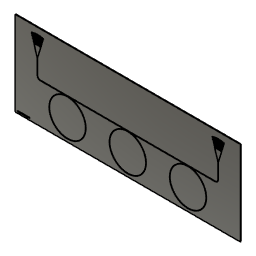
MultiRes (Autodesk Fusion 360 design; units mm, degrees)
Autodesk Fusion 360 part; units mm, degrees
sketch "Sketch1" plane through (0, 0, 0) normal (0, 1, 0) x (1, 0, 0)
  circle A0 centre (0, 0) radius 30
  circle A1 centre (0, 0) radius 30.5
  line L0 (-45, -30.95) -> (45, -30.95)
  line L1 (-50, -35.95) -> (-50, -60.95)
  arc A2 (-45, -30.95) -> (-50, -35.95) centre (-45, -35.95) ccw
  line L2 (-45, -31.2) -> (45, -31.2)
  arc A3 (-45, -31.2) -> (-49.75, -35.95) centre (-45, -35.95) ccw
  line L3 (-49.75, -35.95) -> (-49.75, -60.95)
  line L4 (-45, -30.7) -> (45, -30.7)
  arc A4 (-45, -30.7) -> (-50.25, -35.95) centre (-45, -35.95) ccw
  line L5 (-50.25, -35.95) -> (-50.25, -60.95)
  line L6 (-50.25, -60.95) -> (-49.75, -60.95)
  line L7 (-49.75, -60.95) -> (-39.9666, -92.95)
  line L8 (-50.25, -60.95) -> (-60.0334, -92.95)
  arc A5 (-60.0334, -92.95) -> (-39.9666, -92.95) centre (-50, -60.95) ccw
  arc A6 (-55.6371, -78.5703) -> (-44.3629, -78.5703) centre (-50, -60.95) ccw
  arc A7 (-55.698, -78.7608) -> (-44.302, -78.7608) centre (-50, -60.95) ccw
  arc A8 (-55.7589, -78.9512) -> (-44.2411, -78.9512) centre (-50, -60.95) ccw
  arc A9 (-55.8199, -79.1417) -> (-44.1801, -79.1417) centre (-50, -60.95) ccw
  arc A10 (-55.9722, -79.618) -> (-44.0278, -79.618) centre (-50, -60.95) ccw
  arc A11 (-56.0332, -79.8084) -> (-43.9668, -79.8084) centre (-50, -60.95) ccw
  arc A12 (-56.0941, -79.9989) -> (-43.9059, -79.9989) centre (-50, -60.95) ccw
  arc A13 (-56.1551, -80.1894) -> (-43.8449, -80.1894) centre (-50, -60.95) ccw
  arc A14 (-56.3074, -80.6656) -> (-43.6926, -80.6656) centre (-50, -60.95) ccw
  arc A15 (-56.3683, -80.8561) -> (-43.6317, -80.8561) centre (-50, -60.95) ccw
  arc A16 (-56.4293, -81.0466) -> (-43.5707, -81.0466) centre (-50, -60.95) ccw
  arc A17 (-56.4902, -81.2371) -> (-43.5098, -81.2371) centre (-50, -60.95) ccw
  arc A18 (-56.6426, -81.7133) -> (-43.3574, -81.7133) centre (-50, -60.95) ccw
  arc A19 (-56.7035, -81.9038) -> (-43.2965, -81.9038) centre (-50, -60.95) ccw
  arc A20 (-56.7645, -82.0943) -> (-43.2355, -82.0943) centre (-50, -60.95) ccw
  arc A21 (-56.8254, -82.2848) -> (-43.1746, -82.2848) centre (-50, -60.95) ccw
  arc A22 (-56.9778, -82.761) -> (-43.0222, -82.761) centre (-50, -60.95) ccw
  arc A23 (-57.0387, -82.9515) -> (-42.9613, -82.9515) centre (-50, -60.95) ccw
  arc A24 (-57.0996, -83.142) -> (-42.9004, -83.142) centre (-50, -60.95) ccw
  arc A25 (-57.1606, -83.3325) -> (-42.8394, -83.3325) centre (-50, -60.95) ccw
  arc A26 (-57.3129, -83.8087) -> (-42.6871, -83.8087) centre (-50, -60.95) ccw
  arc A27 (-57.3739, -83.9992) -> (-42.6261, -83.9992) centre (-50, -60.95) ccw
  arc A28 (-57.4348, -84.1897) -> (-42.5652, -84.1897) centre (-50, -60.95) ccw
  arc A29 (-57.4958, -84.3802) -> (-42.5042, -84.3802) centre (-50, -60.95) ccw
  arc A30 (-57.6481, -84.8564) -> (-42.3519, -84.8564) centre (-50, -60.95) ccw
  arc A31 (-57.7091, -85.0469) -> (-42.2909, -85.0469) centre (-50, -60.95) ccw
  arc A32 (-57.77, -85.2374) -> (-42.23, -85.2374) centre (-50, -60.95) ccw
  arc A33 (-57.8309, -85.4279) -> (-42.1691, -85.4279) centre (-50, -60.95) ccw
  arc A34 (-57.9833, -85.9041) -> (-42.0167, -85.9041) centre (-50, -60.95) ccw
  arc A35 (-58.0442, -86.0946) -> (-41.9558, -86.0946) centre (-50, -60.95) ccw
  arc A36 (-58.1052, -86.2851) -> (-41.8948, -86.2851) centre (-50, -60.95) ccw
  arc A37 (-58.1661, -86.4756) -> (-41.8339, -86.4756) centre (-50, -60.95) ccw
  arc A38 (-58.3185, -86.9518) -> (-41.6815, -86.9518) centre (-50, -60.95) ccw
  arc A39 (-58.3794, -87.1423) -> (-41.6206, -87.1423) centre (-50, -60.95) ccw
  arc A40 (-58.4403, -87.3328) -> (-41.5597, -87.3328) centre (-50, -60.95) ccw
  arc A41 (-58.5013, -87.5233) -> (-41.4987, -87.5233) centre (-50, -60.95) ccw
  arc A42 (-58.6536, -87.9995) -> (-41.3464, -87.9995) centre (-50, -60.95) ccw
  arc A43 (-58.7146, -88.19) -> (-41.2854, -88.19) centre (-50, -60.95) ccw
  arc A44 (-58.7755, -88.3805) -> (-41.2245, -88.3805) centre (-50, -60.95) ccw
  arc A45 (-58.8365, -88.571) -> (-41.1635, -88.571) centre (-50, -60.95) ccw
  arc A46 (-58.9888, -89.0472) -> (-41.0112, -89.0472) centre (-50, -60.95) ccw
  arc A47 (-59.0498, -89.2377) -> (-40.9502, -89.2377) centre (-50, -60.95) ccw
  arc A48 (-59.1107, -89.4282) -> (-40.8893, -89.4282) centre (-50, -60.95) ccw
  arc A49 (-59.1716, -89.6186) -> (-40.8284, -89.6186) centre (-50, -60.95) ccw
  arc A50 (-59.324, -90.0949) -> (-40.676, -90.0949) centre (-50, -60.95) ccw
  arc A51 (-59.3849, -90.2854) -> (-40.6151, -90.2854) centre (-50, -60.95) ccw
  arc A52 (-59.4459, -90.4758) -> (-40.5541, -90.4758) centre (-50, -60.95) ccw
  arc A53 (-59.5068, -90.6663) -> (-40.4932, -90.6663) centre (-50, -60.95) ccw
  arc A54 (-59.6592, -91.1426) -> (-40.3408, -91.1426) centre (-50, -60.95) ccw
  arc A55 (-59.7201, -91.333) -> (-40.2799, -91.333) centre (-50, -60.95) ccw
  arc A56 (-59.7811, -91.5235) -> (-40.2189, -91.5235) centre (-50, -60.95) ccw
  arc A57 (-59.842, -91.714) -> (-40.158, -91.714) centre (-50, -60.95) ccw
  arc A58 (-59.9943, -92.1902) -> (-40.0057, -92.1902) centre (-50, -60.95) ccw
  arc A59 (-60.0553, -92.3807) -> (-39.9447, -92.3807) centre (-50, -60.95) ccw
  arc A60 (-60.1162, -92.5712) -> (-39.8838, -92.5712) centre (-50, -60.95) ccw
  arc A61 (-60.1772, -92.7617) -> (-39.8228, -92.7617) centre (-50, -60.95) ccw
  line L9 (-83.2157, 31.3606) -> (-62.7231, 31.3606)
  line L10 (-62.7231, 31.3606) -> (-62.7231, 32.5289)
  line L11 (-62.7231, 32.5289) -> (-83.2157, 32.5289)
  line L12 (-83.2157, 32.5289) -> (-83.2157, 31.3606)
  line L13 (-62.9231, 32.3289) -> (-83.0157, 32.3289)
  line L14 (-83.0157, 32.3289) -> (-83.0157, 31.5606)
  line L15 (-83.0157, 31.5606) -> (-62.9231, 31.5606)
  line L16 (-62.9231, 31.5606) -> (-62.9231, 32.3289)
  line L17 (-73.012, 31.5606) -> (-73.012, 32.3289)
  line L18 (-73.012, 31.5606) -> (-62.9231, 31.5606)
  line L19 (-62.9231, 31.5606) -> (-62.9231, 32.3289)
  line L20 (-62.9231, 32.3289) -> (-73.012, 32.3289)
  line L21 (-73.012, 32.3289) -> (-73.012, 31.5606)
  line L22 (-87.1137, -104.9748) -> (286.8892, -104.9748)
  line L23 (286.8892, -104.9748) -> (286.8892, 35.3192)
  line L24 (286.8892, 35.3192) -> (-87.1137, 35.3192)
  line L25 (-87.1137, 35.3192) -> (-87.1137, -104.9748)
  arc A62 (242.5042, -84.3802) -> (257.4958, -84.3802) centre (250, -60.95) ccw
  arc A63 (243.9668, -79.8084) -> (256.0332, -79.8084) centre (250, -60.95) ccw
  arc A64 (244.302, -78.7608) -> (255.698, -78.7608) centre (250, -60.95) ccw
  arc A65 (243.9059, -79.9989) -> (256.0941, -79.9989) centre (250, -60.95) ccw
  arc A66 (243.2355, -82.0943) -> (256.7645, -82.0943) centre (250, -60.95) ccw
  arc A67 (242.2909, -85.0469) -> (257.7091, -85.0469) centre (250, -60.95) ccw
  arc A68 (243.6317, -80.8561) -> (256.3683, -80.8561) centre (250, -60.95) ccw
  arc A69 (243.6926, -80.6656) -> (256.3074, -80.6656) centre (250, -60.95) ccw
  arc A70 (243.5098, -81.2371) -> (256.4902, -81.2371) centre (250, -60.95) ccw
  arc A71 (242.6261, -83.9992) -> (257.3739, -83.9992) centre (250, -60.95) ccw
  arc A72 (239.9447, -92.3807) -> (260.0553, -92.3807) centre (250, -60.95) ccw
  arc A73 (241.2854, -88.19) -> (258.7146, -88.19) centre (250, -60.95) ccw
  arc A74 (240.5541, -90.4758) -> (259.4459, -90.4758) centre (250, -60.95) ccw
  arc A75 (241.1635, -88.571) -> (258.8365, -88.571) centre (250, -60.95) ccw
  arc A76 (240.2189, -91.5235) -> (259.7811, -91.5235) centre (250, -60.95) ccw
  arc A77 (241.9558, -86.0946) -> (258.0442, -86.0946) centre (250, -60.95) ccw
  arc A78 (242.0167, -85.9041) -> (257.9833, -85.9041) centre (250, -60.95) ccw
  line L26 (249.75, -60.95) -> (239.9666, -92.95)
  line L27 (249.75, -60.95) -> (250.25, -60.95)
  arc A79 (240.3408, -91.1426) -> (259.6592, -91.1426) centre (250, -60.95) ccw
  arc A80 (242.23, -85.2374) -> (257.77, -85.2374) centre (250, -60.95) ccw
  line L28 (250.25, -60.95) -> (260.0334, -92.95)
  arc A81 (240.4932, -90.6663) -> (259.5068, -90.6663) centre (250, -60.95) ccw
  arc A82 (242.1691, -85.4279) -> (257.8309, -85.4279) centre (250, -60.95) ccw
  arc A83 (243.1746, -82.2848) -> (256.8254, -82.2848) centre (250, -60.95) ccw
  arc A84 (244.1801, -79.1417) -> (255.8199, -79.1417) centre (250, -60.95) ccw
  arc A85 (242.6871, -83.8087) -> (257.3129, -83.8087) centre (250, -60.95) ccw
  arc A86 (244.3629, -78.5703) -> (255.6371, -78.5703) centre (250, -60.95) ccw
  arc A87 (243.3574, -81.7133) -> (256.6426, -81.7133) centre (250, -60.95) ccw
  arc A88 (243.8449, -80.1894) -> (256.1551, -80.1894) centre (250, -60.95) ccw
  arc A89 (242.8394, -83.3325) -> (257.1606, -83.3325) centre (250, -60.95) ccw
  arc A90 (240.9502, -89.2377) -> (259.0498, -89.2377) centre (250, -60.95) ccw
  arc A91 (241.6815, -86.9518) -> (258.3185, -86.9518) centre (250, -60.95) ccw
  arc A92 (242.3519, -84.8564) -> (257.6481, -84.8564) centre (250, -60.95) ccw
  arc A93 (242.5652, -84.1897) -> (257.4348, -84.1897) centre (250, -60.95) ccw
  arc A94 (240.676, -90.0949) -> (259.324, -90.0949) centre (250, -60.95) ccw
  arc A95 (244.2411, -78.9512) -> (255.7589, -78.9512) centre (250, -60.95) ccw
  arc A96 (240.6151, -90.2854) -> (259.3849, -90.2854) centre (250, -60.95) ccw
  arc A97 (242.9613, -82.9515) -> (257.0387, -82.9515) centre (250, -60.95) ccw
  arc A98 (239.8228, -92.7617) -> (260.1772, -92.7617) centre (250, -60.95) ccw
  arc A99 (241.8339, -86.4756) -> (258.1661, -86.4756) centre (250, -60.95) ccw
  arc A100 (239.8838, -92.5712) -> (260.1162, -92.5712) centre (250, -60.95) ccw
  arc A101 (242.9004, -83.142) -> (257.0996, -83.142) centre (250, -60.95) ccw
  arc A102 (241.8948, -86.2851) -> (258.1052, -86.2851) centre (250, -60.95) ccw
  arc A103 (243.2965, -81.9038) -> (256.7035, -81.9038) centre (250, -60.95) ccw
  arc A104 (241.2245, -88.3805) -> (258.7755, -88.3805) centre (250, -60.95) ccw
  arc A105 (240.8284, -89.6186) -> (259.1716, -89.6186) centre (250, -60.95) ccw
  arc A106 (240.158, -91.714) -> (259.842, -91.714) centre (250, -60.95) ccw
  arc A107 (240.0057, -92.1902) -> (259.9943, -92.1902) centre (250, -60.95) ccw
  arc A108 (243.0222, -82.761) -> (256.9778, -82.761) centre (250, -60.95) ccw
  arc A109 (239.9666, -92.95) -> (260.0334, -92.95) centre (250, -60.95) ccw
  arc A110 (241.4987, -87.5233) -> (258.5013, -87.5233) centre (250, -60.95) ccw
  arc A111 (244.0278, -79.618) -> (255.9722, -79.618) centre (250, -60.95) ccw
  arc A112 (243.5707, -81.0466) -> (256.4293, -81.0466) centre (250, -60.95) ccw
  arc A113 (241.0112, -89.0472) -> (258.9888, -89.0472) centre (250, -60.95) ccw
  arc A114 (241.5597, -87.3328) -> (258.4403, -87.3328) centre (250, -60.95) ccw
  arc A115 (240.2799, -91.333) -> (259.7201, -91.333) centre (250, -60.95) ccw
  arc A116 (240.8893, -89.4282) -> (259.1107, -89.4282) centre (250, -60.95) ccw
  arc A117 (241.6206, -87.1423) -> (258.3794, -87.1423) centre (250, -60.95) ccw
  arc A118 (241.3464, -87.9995) -> (258.6536, -87.9995) centre (250, -60.95) ccw
  circle A119 centre (100, 0) radius 30.5
  line L29 (55, -30.7) -> (145, -30.7)
  line L30 (55, -30.95) -> (145, -30.95)
  line L31 (55, -31.2) -> (145, -31.2)
  circle A120 centre (100, 0) radius 30
  circle A121 centre (200, 0) radius 30.5
  line L32 (155, -30.7) -> (245, -30.7)
  line L33 (155, -30.95) -> (245, -30.95)
  line L34 (155, -31.2) -> (245, -31.2)
  circle A122 centre (200, 0) radius 30
  line L35 (250, -35.95) -> (250, -60.95)
  line L36 (145, -31.2) -> (155, -31.2)
  line L37 (145, -30.7) -> (155, -30.7)
  line L38 (45, -31.2) -> (55, -31.2)
  line L39 (45, -30.7) -> (55, -30.7)
  arc A123 (250, -35.95) -> (245, -30.95) centre (245, -35.95) ccw
  arc A124 (250.25, -35.95) -> (245, -30.7) centre (245, -35.95) ccw
  line L40 (250.25, -35.95) -> (250.25, -60.95)
  arc A125 (249.75, -35.95) -> (245, -31.2) centre (245, -35.95) ccw
  line L41 (249.75, -35.95) -> (249.75, -60.95)
  point P0 (-50, -30.95)
  point P1 (50, -30.95)
  point P2 (100, 0)
  point P3 (200, 0)
  dimension "d1" = 60
  dimension "d2" = 0.5
  dimension "d3" = 30.95
  dimension "d4" = 50
  dimension "d5" = 50
  dimension "d6" = 30
  dimension "d8" = 5
  dimension "d16" = 107
  dimension "d17" = 107
  dimension "d18" = 32
  dimension "d19" = 32
  dimension "d20" = 18.5
  dimension "d21" = 0.2
  dimension "d22" = 0.4
  dimension "d23" = 0.6
  dimension "d24" = 1.1
  dimension "d25" = 1.3
  dimension "d26" = 1.5
  dimension "d27" = 1.7
  dimension "d28" = 2.2
  dimension "d29" = 2.4
  dimension "d30" = 2.6
  dimension "d31" = 2.8
  dimension "d32" = 3.3
  dimension "d33" = 3.5
  dimension "d34" = 3.7
  dimension "d35" = 3.9
  dimension "d36" = 4.4
  dimension "d37" = 4.6
  dimension "d38" = 4.8
  dimension "d39" = 5
  dimension "d40" = 5.5
  dimension "d41" = 5.7
  dimension "d42" = 5.9
  dimension "d43" = 6.1
  dimension "d44" = 6.6
  dimension "d45" = 6.8
  dimension "d46" = 7
  dimension "d47" = 7.2
  dimension "d48" = 7.7
  dimension "d49" = 7.9
  dimension "d50" = 8.1
  dimension "d51" = 8.3
  dimension "d52" = 8.8
  dimension "d53" = 9
  dimension "d54" = 9.2
  dimension "d55" = 9.4
  dimension "d56" = 9.9
  dimension "d57" = 10.1
  dimension "d58" = 10.3
  dimension "d59" = 10.5
  dimension "d60" = 11
  dimension "d61" = 11.2
  dimension "d62" = 11.4
  dimension "d63" = 11.6
  dimension "d64" = 12.1
  dimension "d65" = 12.3
  dimension "d66" = 12.5
  dimension "d67" = 12.7
  dimension "d68" = 13.2
  dimension "d69" = 13.4
  dimension "d70" = 13.6
  dimension "d71" = 13.8
  dimension "d72" = 14.3
  dimension "d73" = 14.5
  dimension "d74" = 14.7
  dimension "d75" = 14.9
  dimension "d80" = -0.2
  dimension "d88" = 374.0029
  dimension "d89" = 107
  dimension "d90" = 107
  dimension "d91" = 32
  dimension "d92" = 32
  dimension "d95" = 200
  dimension "d96" = 0
  dimension "d97" = 5
  dimension "d98" = 0.25
  dimension "d99" = -0.25
  constraint coincident A0.centre A1.centre
  constraint horizontal L0
  constraint perpendicular L0 L1
  constraint coincident P0 L0
  constraint coincident P0 L1
  constraint tangent L0 A2
  constraint tangent L1 A2
  constraint coincident P1 L0
  constraint perpendicular L3 L6
  constraint coincident L1.end A5.centre
  constraint coincident L8 A6.start
  constraint coincident L7 A6.end
  constraint horizontal L9
  constraint vertical L10
  constraint horizontal L11
  constraint vertical L12
  constraint coincident L15 L17.start
  constraint coincident L13 L17.end
  constraint perpendicular L13 L17
  constraint horizontal L18
  constraint vertical L19
  constraint horizontal L20
  constraint vertical L21
  constraint horizontal L22
  constraint vertical L23
  constraint horizontal L24
  constraint vertical L25
  constraint concentric A2 A4
  constraint tangent L4 A4
  constraint tangent A4 L5
  constraint concentric A2 A3
  constraint tangent L2 A3
  constraint tangent A3 L3
  constraint coincident A62.centre A63.centre
  constraint perpendicular L27 L35
  constraint tangent L35 A123
  constraint coincident L33.end A123.end
  measures "d1" diameter of A0
  measures "d3" distance of A0.centre L0
  measures "d4" horizontal distance of A0.centre P1
  measures "d5" horizontal distance of A0.centre P0
  measures "d6" distance of P0 L1.end
  measures "d8" radius of A2
  measures "d16" angle of L6 L8
  measures "d17" angle of L6 L7
  measures "d18" vertical distance of L3.end L7.end
  measures "d19" vertical distance of L5.end L8.end
  measures "d20" radius of A6
  measures "d88" distance of L22.start L22.end
  measures "d89" angle of L27 L28
  measures "d90" angle of L26 L27
  measures "d91" vertical distance of L28.end L27.end
  measures "d92" vertical distance of L26.end A62.centre
  measures "d97" radius of A123
extrude "Extrude1" add sketch "Sketch1" against normal blind 0.22 contours A1 | L2 A3 L3 L4 A4 L5 L6 L27 L29 L31 L32 L34 L36 L37 L38 L39 A124 L40 A125 L41 | L6 L7 L8 A6 | L7 L8 A7 A8 | L7 L8 A9 A10 | L26 L27 L28 A86 | L7 L8 A11 A12 | A64 L26 L28 A95 | L7 L8 A13 A14 | L26 L28 A84 A111 | L7 L8 A15 A16 | A63 A65 L26 L28 | L7 L8 A17 A18 | A69 L26 L28 A88 | L7 L8 A19 A20 | A68 L26 L28 A112 | L7 L8 A21 A22 | A70 L26 L28 A87 | L7 L8 A23 A24 | A66 L26 L28 A103 | L7 L8 A25 A26 | L26 L28 A83 A108 | L7 L8 A27 A28 | L26 L28 A97 A101 | L7 L8 A29 A30 | L26 L28 A85 A89 | L7 L8 A31 A32 | A71 L26 L28 A93 | L7 L8 A33 A34 | A62 L26 L28 A92 | L7 L8 A35 A36 | A67 L26 A80 L28 | L7 L8 A37 A38 | A78 L26 L28 A82 | L7 L8 A39 A40 | A77 L26 L28 A102 | L7 L8 A41 A42 | L26 L28 A91 A99 | L7 L8 A43 A44 | L26 L28 A114 A117 | L7 L8 A45 A46 | L26 L28 A110 A118 | L7 L8 A47 A48 | A73 L26 L28 A104 | L7 L8 A49 A50 | A75 L26 L28 A113 | L7 L8 A51 A52 | L26 L28 A90 A116 | L7 L8 A53 A54 | L26 L28 A94 A105 | L7 L8 A55 A56 | A74 L26 L28 A96 | L7 L8 A57 A58 | L26 A79 L28 A81 | L7 L8 A59 A60 | A76 L26 L28 A115 | L7 L8 A5 A61 | L26 L28 A106 A107 | A72 L26 L28 A100 | L26 L28 A98 A109 | L9 L10 L11 L12 | L13 L14 L15 L17 L21 | A119 | A121 makes body 1 at (-58.3639, -0.0733, 91.9412) makes body 2 at (-56.6256, -0.1467, 90.1067) makes body 3 at (-56.1507, -0.1467, 87.9585) makes body 4 at (-52.5972, -0.1467, 86.3174) makes body 5 at (-43.8742, -0.1467, 83.4303) makes body 6 at (-52.1627, -0.1467, 81.9389) makes body 7 at (-51.9455, -0.1467, 79.7496) makes body 8 at (-79.8145, 0, -32.0728) makes body 9 at (-45.6353, 0, 79.8529) makes body 10 at (-45.1612, 0, 81.9978) makes body 11 at (-55.313, 0, 84.1426) makes body 12 at (-55.7871, 0, 86.2875) makes body 13 at (-56.2613, 0, 88.4323) makes body 14 at (-56.7354, 0, 90.5771) makes body 15 at (-49.3456, 0, 93.523) makes body 16 at (-58.7291, -0.0733, 93.3301) makes body 17 at (-49.3673, 0, 92.425) makes body 18 at (-43.5017, 0, 89.5047) makes body 19 at (-56.0242, 0, 87.3599) makes body 20 at (-55.5501, 0, 85.2151) makes body 21 at (-44.9241, 0, 83.0702) makes body 22 at (-54.6018, 0, 80.9254) makes body 23 at (250.6544, 0, 93.523) makes body 24 at (-21.122, 0, 21.6654) makes body 25 at (-47.1291, -0.1467, 80.7429) makes body 26 at (-46.8255, -0.1467, 82.9219) makes body 27 at (-52.4886, -0.1467, 85.2228) makes body 28 at (-56.9651, -0.0733, 86.6219) makes body 29 at (-52.923, -0.1467, 89.6013) makes body 30 at (-53.1403, -0.1467, 91.7905) makes body 31 at (-53.3575, -0.1467, 93.9798) makes body 32 at (256.7354, 0, 90.5771) makes body 33 at (256.2613, 0, 88.4323) makes body 34 at (255.7871, 0, 86.2875) makes body 35 at (244.687, 0, 84.1426) makes body 36 at (254.8388, 0, 81.9978) makes body 37 at (254.3647, 0, 79.8529) makes body 38 at (248.0545, -0.1467, 79.7496) makes body 39 at (253.0227, -0.1467, 81.8324) makes body 40 at (250.4768, -0.1467, 84.2451) makes body 41 at (243.3147, -0.0733, 85.558) makes body 42 at (247.1856, -0.1467, 88.5067) makes body 43 at (243.3744, -0.1467, 90.1067) makes body 44 at (245.4591, -0.0733, 92.7272) makes body 45 at (245.3072, -0.0733, 93.8167) makes body 46 at (254.3891, -0.1467, 91.6377) makes body 47 at (247.077, -0.1467, 89.6013) makes body 48 at (247.2942, -0.1467, 87.412) makes body 49 at (250.4985, -0.1467, 85.3449) makes body 50 at (253.1745, -0.1467, 82.9219) makes body 51 at (247.9459, -0.1467, 80.8442) makes body 52 at (129.3238, 0, 7.4595) makes body 53 at (249.9167, 0, 73.2597) makes body 54 at (172.1155, 0, -11.7467) makes body 55 at (254.6018, 0, 80.9254) makes body 56 at (244.9241, 0, 83.0702) makes body 57 at (244.4499, 0, 85.2151) makes body 58 at (256.0242, 0, 87.3599) makes body 59 at (243.5017, 0, 89.5047) makes body 60 at (250.6327, 0, 92.425) makes body 61 at (245.2608, -0.0733, 94.1495)
extrude "Extrude2" add sketch "Sketch1" along normal blind 1 separate body contours A0 | A1 | L2 A3 L3 L4 A4 L5 L6 L27 L29 L31 L32 L34 L36 L37 L38 L39 A124 L40 A125 L41 | L6 L7 L8 A6 | L7 L8 A6 A7 | L7 L8 A7 A8 | L7 L8 A8 A9 | L7 L8 A9 A10 | L26 L27 L28 A86 | L7 L8 A10 A11 | A64 L26 L28 A86 | L7 L8 A11 A12 | A64 L26 L28 A95 | L7 L8 A12 A13 | L26 L28 A84 A95 | L7 L8 A13 A14 | L26 L28 A84 A111 | L7 L8 A14 A15 | A63 L26 L28 A111 | L7 L8 A15 A16 | A63 A65 L26 L28 | L7 L8 A16 A17 | A65 L26 L28 A88 | L7 L8 A17 A18 | A69 L26 L28 A88 | L7 L8 A18 A19 | A68 A69 L26 L28 | L7 L8 A19 A20 | A68 L26 L28 A112 | L7 L8 A20 A21 | A70 L26 L28 A112 | L7 L8 A21 A22 | A70 L26 L28 A87 | L7 L8 A22 A23 | L26 L28 A87 A103 | L7 L8 A23 A24 | A66 L26 L28 A103 | L7 L8 A24 A25 | A66 L26 L28 A83 | L7 L8 A25 A26 | L26 L28 A83 A108 | L7 L8 A26 A27 | L26 L28 A97 A108 | L7 L8 A27 A28 | L26 L28 A97 A101 | L7 L8 A28 A29 | L26 L28 A89 A101 | L7 L8 A29 A30 | L26 L28 A85 A89 | L7 L8 A30 A31 | A71 L26 L28 A85 | L7 L8 A31 A32 | A71 L26 L28 A93 | L7 L8 A32 A33 | A62 L26 L28 A93 | L7 L8 A33 A34 | A62 L26 L28 A92 | L7 L8 A34 A35 | A67 L26 L28 A92 | L7 L8 A35 A36 | A67 L26 A80 L28 | L7 L8 A36 A37 | L26 A80 L28 A82 | L7 L8 A37 A38 | A78 L26 L28 A82 | L7 L8 A38 A39 | A77 A78 L26 L28 | L7 L8 A39 A40 | A77 L26 L28 A102 | L7 L8 A40 A41 | L26 L28 A99 A102 | L7 L8 A41 A42 | L26 L28 A91 A99 | L7 L8 A42 A43 | L26 L28 A91 A117 | L7 L8 A43 A44 | L26 L28 A114 A117 | L7 L8 A44 A45 | L26 L28 A110 A114 | L7 L8 A45 A46 | L26 L28 A110 A118 | L7 L8 A46 A47 | A73 L26 L28 A118 | L7 L8 A47 A48 | A73 L26 L28 A104 | L7 L8 A48 A49 | A75 L26 L28 A104 | L7 L8 A49 A50 | A75 L26 L28 A113 | L7 L8 A50 A51 | L26 L28 A90 A113 | L7 L8 A51 A52 | L26 L28 A90 A116 | L7 L8 A52 A53 | L26 L28 A105 A116 | L7 L8 A53 A54 | L26 L28 A94 A105 | L7 L8 A54 A55 | L26 L28 A94 A96 | L7 L8 A55 A56 | A74 L26 L28 A96 | L7 L8 A56 A57 | A74 L26 L28 A81 | L7 L8 A57 A58 | L26 A79 L28 A81 | L7 L8 A58 A59 | L26 A79 L28 A115 | L7 L8 A59 A60 | A76 L26 L28 A115 | L7 L8 A60 A61 | A76 L26 L28 A106 | L7 L8 A5 A61 | L26 L28 A106 A107 | A72 L26 L28 A107 | A72 L26 L28 A100 | L26 L28 A98 A100 | L26 L28 A98 A109 | L9 L10 L11 L12 | L13 L15 L16 L17 L18 L19 L20 L21 | L13 L14 L15 L17 L21 | L22 L23 L24 L25 | A119 | A120 | A121 | A122 makes body 62
sketch "Sketch2" plane through (0, 0, 0) normal (0, -1, 0) x (1, 0, 0)
  line L0 (-87.1137, 104.9748) -> (-87.1137, -35.3192)
  line L1 (-87.1137, -35.3192) -> (286.8892, -35.3192)
  line L2 (286.8892, -35.3192) -> (286.8892, 104.9748)
  line L3 (286.8892, 104.9748) -> (-87.1137, 104.9748)
  line L4 (-69.5, -30.5) -> (-62.7446, -30.5)
  line L5 (-69.1517, -30.5) -> (-62.7712, -30.5) construction
  line L6 (-62.7712, -30.5) -> (-62.7712, -28.788) construction
  line L7 (-62.7712, -28.788) -> (-69.1517, -28.788) construction
  line L8 (-69.1517, -28.788) -> (-69.1517, -30.5) construction
  dimension "d85" = 1.6
  text T0 "20 μm" font "Arial" height 1.6 align left top in box 6.3805 x 1.712 at (-69.1517, -30.5) x (1, 0) y (0, 1) spacing 1 kerned
  constraint horizontal L4
  constraint coincident L4
extrude "Extrude3" add sketch "Sketch2" along normal blind 0.22 separate body text T0 makes body 63 at (-67.7443, 0, -29.7391) makes body 64 at (-65.8716, 0, -29.9852) makes body 65 at (-64.6113, 0, -29.8012) makes body 66 at (-68.708, 0, -30.3251)
equation "d3 = 30 mm + 0.5 mm + 0.2 mm + 0.25 mm"
equation "d24 = 0.6 mm + 0.5 mm"
equation "d88 = 174.0029105048 mm + 100 mm + 100 mm"
named bodies: "Escala", "Base"
